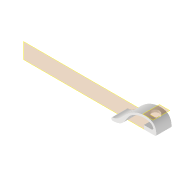
# Autodesk Inventor part: 30_XYTabel_Aliexpress_cellSTORM_chiptray_clamp
Saved by Autodesk Inventor 2022 (Build 260153000, 153)
## iProperties
Created: 2022-01-03
Part Number: 30_XYTabel_Aliexpress_cellSTORM_chiptray_clamp
Material: Generisch
Document SubType Name: Modeling
Designer: diederichbenedict
Density: 1 g/cm^3
Appearance: Vorgabe
Author: diederichbenedict
Autodesk Inventor part; units mm, degrees
ref_plane "YZ Plane" through (0, 0, 0) normal (1, 0, 0) x (0, 1, 0)
ref_plane "XZ Plane" through (0, 0, 0) normal (0, 1, 0) x (-1, 0, 0)
ref_plane "XY Plane" through (0, 0, 0) normal (0, 0, 1) x (1, 0, 0)
ref_plane "Arbeitsebene1" through (0, 0, 0) normal (0, 0, 1) x (1, 0, 0)
sketch "Skizze1" plane through (0, 0, 0) normal (0, 0, 1) x (1, 0, 0)
  line L0 (78, 3) -> (108.3, 3) projected
  line L1 (77, -2.3955) -> (1, -2.3955) projected
  line L2 (88.6, 3) -> (91.4, 3) projected
  line L3 (91.4, 3) -> (91.4, 0)
  line L4 (88.6, 3) -> (88.6, 0)
  line L5 (83.7973, 3) -> (93.4, 3)
  line L6 (93.4, 3) -> (93.4, 8.7752) construction
  line L7 (93.4, 8.7752) -> (89.9261, 12.2491) construction
  line L8 (89.9261, 12.2491) -> (75.4775, 12.2491) construction
  line L9 (75.4775, 12.2491) -> (69.5721, -0.415) construction
  line L10 (69.5721, -0.415) -> (65.4051, -0.415) construction
  line L11 (65.4051, -0.415) -> (63.7727, -0.415) construction
  spline S0 degree 4 poles (93.4, 3) (93.4, 8.7752) (89.9261, 12.2491) (75.4775, 12.2491) (69.5721, -0.415) (65.4051, -0.415) (63.7727, -0.415) knots 1 1 1 1 1 2 3 4 4 4 4 4
  line L12 (91.4, 5.5) -> (91.4, 7.9468) construction
  line L13 (91.4, 7.9468) -> (89.0977, 10.2491) construction
  line L14 (89.0977, 10.2491) -> (76.7516, 10.2491) construction
  line L15 (76.7516, 10.2491) -> (73.2926, 2.8311) construction
  line L16 (73.2926, 2.8311) -> (70.8463, -2.415) construction
  line L17 (70.8463, -2.415) -> (63.7727, -2.415) construction
  spline S1 degree 4 poles (91.4, 5.5) (91.4, 7.9468) (89.0977, 10.2491) (76.7516, 10.2491) (73.2926, 2.8311) (70.8463, -2.415) (63.7727, -2.415) knots 1 1 1 1 1 2 3 4 4 4 4 4
  line L18 (91.4, 5.5) -> (83.7973, 5.5)
  line L19 (83.7973, 5.5) -> (83.7973, 3)
  line L20 (63.7727, -2.415) -> (63.7727, -0.415)
  point P0 (0, 0)
  point P1 (63.7727, -2.3955)
  point P2 (64.7379, -2.3955)
  dimension "d0" = 2
  dimension "d1" = 2
  dimension "d2" = 2
  dimension "d3" = 2
  dimension "d4" = 2
  dimension "d5" = 45
  dimension "d6" = 65
  dimension "d7" = 2.5
  constraints: 12 end point, 7 parallel, 4 vertical, 2 collinear, 2 perpendicular, 2 point on line, 8 other
  measures "d0" distance between parallel lines of L13 L7
  measures "d1" distance between parallel lines of L14 L8
  measures "d2" distance between parallel lines of L9 L15
  measures "d3" distance between parallel lines of L11 L17
  measures "d4" distance between parallel lines of L6 L12
  measures "d5" angle of L0 L7
  measures "d6" angle of L0 L9
  measures "d7" distance between parallel lines of L5 L18
extrude "Extrusion1" add sketch "Skizze1" along normal blind 10 contours L19 L18 S1 L1 L20 S0 L0
ref_plane "Arbeitsebene2" through (83.7973, 11.75, 0) normal (0, 1, 0) x (1, 0, 0)
sketch "Skizze2" plane through (83.7973, 11.75, 0) normal (0, 1, 0) x (1, 0, 0)
  line L0 (7.6027, 0) -> (0, 0) projected
  line L1 (0, 0) -> (0, -10) projected
  line L2 (7.6027, -10) -> (0, -10) projected
  line L3 (7.6027, 0) -> (7.6027, -10) projected
  circle A0 centre (2.6244, -5) radius 1
  point P0 (-83.7973, 0)
  dimension "d11" = 2
  constraints: 1 centre point
  measures "d11" diameter of A0
hole "Bohrung1" at (86.4217, 11.75, 5) direction (0, -1, 0) diameter 2.8 end through all counterbore diameter 5.5 counterbore depth 5
fillet "Rundung1" radius 1 4 edges at (91.4, 5.5, 5) (63.7727, -0.415, 5) (63.7727, -2.3955, 5) (93.4, 3, 5)
